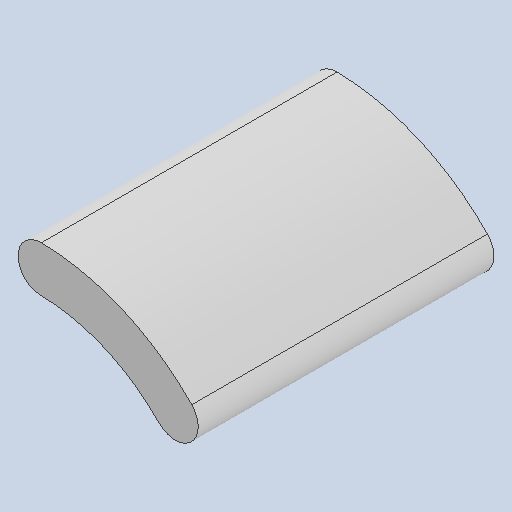
# Autodesk Inventor part: Clutch_Pin
Saved by Autodesk Inventor 2024.3 (Build 283343000, 343)
## iProperties
Created: 2024-11-08
Part Number: Clutch_Pin
Material: Generic
Document SubType Name: Modeling
Designer: wszaf
Density: 1 g/cm^3
Appearance: Default
Author: wszaf
Autodesk Inventor part; units mm, degrees
ref_plane "YZ Plane" through (0, 0, 0) normal (1, 0, 0) x (0, 1, 0)
ref_plane "XZ Plane" through (0, 0, 0) normal (0, 1, 0) x (-1, 0, 0)
ref_plane "XY Plane" through (0, 0, 0) normal (0, 0, 1) x (1, 0, 0)
sketch "Sketch1" plane through (0, 0, 0) normal (0, 0, 1) x (1, 0, 0)
  arc A0 (-6.0322, -5.8457) -> (-0.1319, -8.399) centre (0, 0) ccw projected
  arc A1 (-0.1319, -8.399) -> (-0.1036, -6.5992) centre (-0.1178, -7.4991) ccw projected
  arc A2 (-4.7396, -4.593) -> (-0.1036, -6.5992) centre (0, 0) ccw projected
  arc A3 (-4.7396, -4.593) -> (-6.0322, -5.8457) centre (-5.3859, -5.2194) ccw projected
  arc A4 (5.8457, -6.0322) -> (8.399, -0.1319) centre (0, 0) ccw projected
  arc A5 (8.399, -0.1319) -> (6.5992, -0.1036) centre (7.4991, -0.1178) ccw projected
  arc A6 (4.593, -4.7396) -> (6.5992, -0.1036) centre (0, 0) ccw projected
  arc A7 (4.593, -4.7396) -> (5.8457, -6.0322) centre (5.2194, -5.3859) ccw projected
  arc A8 (6.0322, 5.8457) -> (0.1319, 8.399) centre (0, 0) ccw projected
  arc A9 (0.1319, 8.399) -> (0.1036, 6.5992) centre (0.1178, 7.4991) ccw projected
  arc A10 (4.7396, 4.593) -> (0.1036, 6.5992) centre (0, 0) ccw projected
  arc A11 (4.7396, 4.593) -> (6.0322, 5.8457) centre (5.3859, 5.2194) ccw projected
  arc A12 (-5.8457, 6.0322) -> (-8.399, 0.1319) centre (0, 0) ccw projected
  arc A13 (-8.399, 0.1319) -> (-6.5992, 0.1036) centre (-7.4991, 0.1178) ccw projected
  arc A14 (-4.593, 4.7396) -> (-6.5992, 0.1036) centre (0, 0) ccw projected
  arc A15 (-4.593, 4.7396) -> (-5.8457, 6.0322) centre (-5.2194, 5.3859) ccw projected
  circle A16 centre (0, 0) radius 9 projected
  circle A17 centre (0, 0) radius 6 projected
  point P0 (0, 0)
extrude "Extrusion1" add sketch "Sketch1" along normal blind 11.6 contours A11 A10 A9 A8
equation "\"Fit_Loose\" = 0.4"
body "Solid1"
